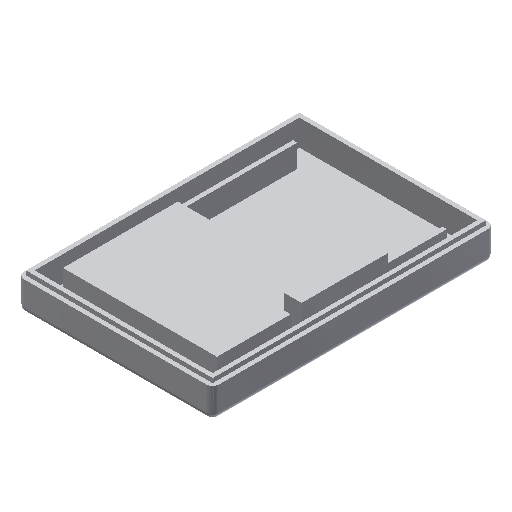
# Autodesk Inventor part: superior
Saved by Autodesk Inventor 2025.2 (Build 292293000, 293)
## iProperties
Created: 2025-10-19
Part Number: superior
Material: ABS Plastic
Document SubType Name: Sheet Metal
Designer: Ricardo
Density: 1.06 g/cm^3
Sheet Metal Rule: Default_mm
Appearance: Smooth - White
Mass: 10.1379 g
Surface Area: 106.906 cm^2
Volume: 9.56404 cm^3
Author: Ricardo
Autodesk Inventor part; units mm, degrees
ref_plane "YZ Plane" through (0, 0, 0) normal (1, 0, 0) x (0, 1, 0)
ref_plane "XZ Plane" through (0, 0, 0) normal (0, 1, 0) x (-1, 0, 0)
ref_plane "XY Plane" through (0, 0, 0) normal (0, 0, 1) x (1, 0, 0)
sketch "Sketch1" plane through (0, 0, 0) normal (0, 1, 0) x (-1, 0, 0)
  line L0 (0, 0) -> (45, 0)
  line L1 (45, 0) -> (45, -65)
  line L2 (45, -65) -> (0, -65)
  line L3 (0, -65) -> (0, 0)
  dimension "d0" = 45
  dimension "d1" = 65
  constraints: 8 end point, 2 parallel, 1 horizontal, 1 perpendicular
  measures "d0" distance of L1.end L2.end
  measures "d1" distance of L0.end L1.end
extrude "Extrusion1" add sketch "Sketch1" along normal blind 2
sketch "Sketch2" plane through (0, 2, 0) normal (0, 1, 0) x (1, 0, 0)
  line L0 (0, 65) -> (0, 0) projected
  line L1 (0, 0) -> (-45, 0) projected
  line L2 (-45, 0) -> (-45, 65) projected
  line L3 (-45, 65) -> (0, 65) projected
  line L4 (-45, 0) -> (0, 0) projected
  line L5 (-45, 65) -> (-45, 0) projected
  line L6 (0, 65) -> (-45, 65) projected
  line L7 (0, 0) -> (0, 65) projected
  line L8 (-2, 2) -> (-43, 2)
  line L9 (-43, 2) -> (-43, 63)
  line L10 (-43, 63) -> (-2, 63)
  line L11 (-2, 63) -> (-2, 2)
  dimension "d4" = 2
  dimension "d5" = 2
  dimension "d6" = 2
  dimension "d7" = 2
  constraints: 8 end point, 2 parallel, 1 horizontal, 1 perpendicular
  measures "d4" distance between parallel lines of L2 L9
  measures "d5" distance between parallel lines of L0 L11
  measures "d6" distance between parallel lines of L3 L10
  measures "d7" distance between parallel lines of L1 L8
extrude "Extrusion2" add sketch "Sketch2" along normal blind 2
sketch "Sketch3" plane through (0, 2, 0) normal (0, 1, 0) x (1, 0, 0)
  line L0 (-5.5, 6.5) -> (-39, 6.5)
  line L1 (-39, 6.5) -> (-39, 57.5)
  line L2 (-39, 57.5) -> (-5.5, 57.5)
  line L3 (-5.5, 57.5) -> (-5.5, 6.5)
  line L4 (0, 0) -> (0, 65) construction
  line L5 (0, 32.5) -> (-39, 32.5) construction
  line L6 (-45, 0) -> (0, 0) construction
  line L7 (-22.5, 0) -> (-22.5, 65) construction
  line L8 (0, 65) -> (-45, 65) construction
  line L9 (-4.5, 58.5) -> (-40, 58.5)
  line L10 (-40, 58.5) -> (-40, 5.5)
  line L11 (-40, 5.5) -> (-4.5, 5.5)
  line L12 (-4.5, 5.5) -> (-4.5, 58.5)
  line L13 (-2, 2) -> (-2, 63) projected
  line L14 (-2, 63) -> (-43, 63) projected
  line L15 (-43, 63) -> (-43, 2) projected
  line L16 (-43, 2) -> (-2, 2) projected
  line L17 (0, 65) -> (0, 0) projected
  line L18 (0, 0) -> (-45, 0) projected
  line L19 (-45, 0) -> (-45, 65) projected
  line L20 (-45, 65) -> (0, 65) projected
  dimension "d10" = 33.5
  dimension "d11" = 51
  dimension "d12" = 26
  dimension "d13" = 17
  dimension "d14" = 1
  dimension "d15" = 1
  dimension "d16" = 1
  dimension "d17" = 1
  dimension "d25" = 51
  constraints: 20 end point, 4 parallel, 3 midpoint, 3 perpendicular, 2 horizontal, 1 point on line
  measures "d10" distance of L1.end L2.end
  measures "d11" distance of L2.end L0.start
  measures "d12" distance between parallel lines of L0 L5
  measures "d13" distance between parallel lines of L7 L3
  measures "d14" distance between parallel lines of L3 L12
  measures "d15" distance between parallel lines of L11 L0
  measures "d16" distance between parallel lines of L1 L10
  measures "d17" distance between parallel lines of L2 L9
  measures "d25" distance of L0.end L1.end
extrude "Extrusion3" add sketch "Sketch3" along normal blind 5.25 contours L12 L11 L10 L9
sketch "Sketch4" plane through (-4.5, 2, -58.5) normal (0, 0, -1) x (-1, 0, 0)
  line L0 (35.5, 0) -> (0, 0) projected
  line L1 (35.5, 0) -> (35.5, 5.25) projected
  line L2 (0, 5.25) -> (35.5, 5.25) projected
  line L3 (0, 0) -> (0, 5.25) projected
  line L4 (1, 5.25) -> (34.5, 5.25)
  line L5 (34.5, 5.25) -> (34.5, 0)
  line L6 (34.5, 0) -> (1, 0)
  line L7 (1, 0) -> (1, 5.25)
  point P0 (-4.5, -2)
  point P1 (1, 0)
  point P2 (34.5, 0)
  dimension "d20" = 1
  dimension "d21" = 1
  dimension "d22" = 0
  constraints: 8 end point, 2 parallel, 1 horizontal, 1 perpendicular, 1 point on line
  measures "d20" distance between parallel lines of L3 L7
  measures "d21" distance between parallel lines of L1 L5
  measures "d22" distance between parallel lines of L0 L6
extrude "Extrusion4" cut sketch "Sketch4" against normal blind 2 contours L0 L7 L2 L5
sketch "Sketch5" plane through (0, 7.25, 0) normal (0, 1, 0) x (1, 0, 0)
  line L0 (-39, 58.5) -> (-39, 6.5) projected
  line L1 (-39, 6.5) -> (-5.5, 6.5) projected
  line L2 (-5.5, 6.5) -> (-5.5, 58.5) projected
  line L3 (-5.5, 58.5) -> (-4.5, 58.5) projected
  line L4 (-4.5, 58.5) -> (-4.5, 5.5) projected
  line L5 (-4.5, 5.5) -> (-40, 5.5) projected
  line L6 (-40, 5.5) -> (-40, 58.5) projected
  line L7 (-40, 58.5) -> (-39, 58.5) projected
  line L8 (-40, 5.5) -> (-4.5, 5.5)
  line L9 (-4.5, 5.5) -> (-4.5, 32)
  line L10 (-4.5, 32) -> (-40, 32)
  line L11 (-40, 32.75) -> (-40, 5.5)
  line L12 (-4.5, 32) -> (-40, 32)
  line L13 (-40, 32) -> (-40, 5.5)
  line L14 (-40, 5.5) -> (-4.5, 5.5)
  line L15 (-4.5, 5.5) -> (-4.5, 32)
  line L16 (-40, 58.5) -> (-40, 5.5) projected
  line L17 (-40, 5.5) -> (-4.5, 5.5) projected
  line L18 (-4.5, 5.5) -> (-4.5, 58.5) projected
  line L19 (-4.5, 32) -> (-40, 32)
  line L20 (-40, 32) -> (-40, 5.5)
  line L21 (-40, 5.5) -> (-4.5, 5.5)
  line L22 (-4.5, 5.5) -> (-4.5, 32.75)
  point P0 (0, 0)
  point P1 (-5.5, 32)
  point P2 (-39, 32)
  constraints: 24 end point, 5 parallel, 3 perpendicular, 2 horizontal, 1 midpoint
extrude "Extrusion6" add sketch "Sketch5" along normal blind 1 contours L10 L2 L1 L0 | L0 L1 L2 L10 L4 L5 L6
fillet "Fillet1" radius 1.5 1 edges at (-22.5, 0, 0)
fillet "Fillet2" radius 1.5 1 edges at (-22.5, 0, -65)
sketch "Sketch13" plane through (0, 8.25, 0) normal (0, 1, 0) x (1, 0, 0)
  line L0 (0, 0) -> (0, 65) projected
  line L1 (-4.5, 5.5) -> (-4.5, 32) projected
  line L2 (-4.5, 32) -> (-4.5, 58.5) projected
  line L3 (-5.5, 6.5) -> (-5.5, 58.5) projected
  line L4 (-40, 32) -> (-40, 5.5) construction
  line L5 (-40, 5.5) -> (-4.5, 5.5) construction
  line L6 (-4.5, 5.5) -> (-4.5, 32) construction
  line L7 (-4.5, 32) -> (-40, 32) construction
  line L8 (-2, 63) -> (-2, 2) projected
  line L9 (-40, 5.5) -> (-4.5, 5.5) projected
  line L10 (-4.5, 32) -> (-40, 32) projected
  line L11 (-2, 42.5) -> (-6, 42.5)
  line L12 (-6, 42.5) -> (-6, 22.5)
  line L13 (-6, 22.5) -> (-2, 22.5)
  line L14 (-2, 22.5) -> (-2, 42.5)
  line L15 (-2, 2) -> (-43, 2) projected
  point P0 (-5.75, 59.75)
  point P1 (-4.5, 22.5)
  point P2 (-2, 22.5)
  point P3 (-4.5, 42.5)
  dimension "d58" = 4
  dimension "d59" = 20
  dimension "d60" = 20.5
  constraints: 8 end point, 2 parallel, 1 horizontal, 1 perpendicular, 1 point on line, 1 other
  measures "d58" distance of L13.end L12.end
  measures "d59" distance of L11.end L12.end
  measures "d60" distance between parallel lines of L15 L13
extrude "Extrusion12" add sketch "Sketch13" along normal mid plane 7
sketch "Sketch15" plane through (-2, 11.75, -42.5) normal (0, 0, -1) x (-1, 0, 0)
  line L0 (4, -3.5) -> (38, -3.5) projected
  line L1 (4, -4.5) -> (37, -4.5) projected
  line L2 (3.5, -7) -> (3.5, -4.5) projected
  line L3 (37, -9.75) -> (3.5, -9.75) projected
  line L4 (3.5, -4.5) -> (4, -4.5)
  line L5 (4, -4.5) -> (4, -13.75)
  line L6 (4, -13.75) -> (3.5, -13.75)
  line L7 (3.5, -13.75) -> (3.5, -4.5)
  point P0 (-2, -11.75)
  point P1 (3.5, -13.75)
  point P2 (4, -9.75)
  constraints: 8 end point, 2 parallel, 1 horizontal, 1 perpendicular, 1 other
extrude "Extrusion14" cut sketch "Sketch15" against normal up to surface (36 mm away) contours L2 L4 L5 L3 L7
sketch "Sketch16" plane through (0, 4, 0) normal (0, 1, 0) x (1, 0, 0)
  line L0 (-2, 22.5) -> (-2, 42.5) projected
  line L1 (-2, 22.5) -> (-2, 2) projected
  line L2 (-2, 2) -> (-43, 2) projected
  line L3 (-45, 0) -> (0, 0) projected
  line L4 (0, 0) -> (0, 65) projected
  line L5 (-2, 63) -> (-2, 42.5) projected
  line L6 (-43, 63) -> (-2, 63) projected
  line L7 (0, 65) -> (-45, 65) projected
  line L8 (-45, 65) -> (-45, 0) projected
  line L9 (-43, 2) -> (-43, 63) projected
  line L10 (0, 65) -> (-45, 65)
  line L11 (-45, 65) -> (-45, 0)
  line L12 (-45, 0) -> (0, 0)
  line L13 (0, 0) -> (0, 65)
  line L14 (-43, 2) -> (-2, 2)
  line L15 (-2, 2) -> (-2, 63)
  line L16 (-2, 63) -> (-43, 63)
  line L17 (-43, 63) -> (-43, 2)
  constraints: 16 end point, 4 parallel, 2 horizontal, 2 perpendicular
extrude "Extrusion15" add sketch "Sketch16" along normal blind 4
sketch "Sketch17" plane through (0, 8, 0) normal (0, 1, 0) x (1, 0, 0)
  line L0 (0, 0) -> (0, 65) projected
  line L1 (0, 65) -> (-45, 65) projected
  line L2 (-45, 0) -> (0, 0) projected
  line L3 (-45, 65) -> (-45, 0) projected
  line L4 (-1, 64) -> (-44, 64)
  line L5 (-44, 64) -> (-44, 1)
  line L6 (-44, 1) -> (-1, 1)
  line L7 (-1, 1) -> (-1, 64)
  dimension "d71" = 1
  dimension "d72" = 1
  dimension "d73" = 1
  dimension "d74" = 1
  constraints: 8 end point, 2 parallel, 1 horizontal, 1 perpendicular
  measures "d71" distance between parallel lines of L2 L6
  measures "d72" distance between parallel lines of L0 L7
  measures "d73" distance between parallel lines of L1 L4
  measures "d74" distance between parallel lines of L5 L3
extrude "Extrusion16" cut sketch "Sketch17" against normal blind 1
fillet "Fillet3" radius 1.5 5 edges at (0, 0.4393, -0.4393) (0, 0, -32.5) (0, 0.4393, -64.5607) (0, 4.25, -65) (0, 4.25, 0)
fillet "Fillet4" radius 1.5 5 edges at (-45, 0.4393, -0.4393) (-45, 4.25, 0) (-45, 0.4393, -64.5607) (-45, 4.25, -65) (-45, 0, -32.5)
equation "\"BendRadius\" = Thickness"
equation "\"BendReliefWidth\" = Thickness"
equation "\"BendReliefDepth\" = 0.5 * Thickness"
equation "\"CornerReliefSize\" = 4 * Thickness"
equation "\"MinimumRemnant\" = 2 * Thickness"
equation "\"TransitionRadius\" = BendRadius"
equation "\"JacobiRadiusSize\" = BendRadius"
equation "\"GapSize\" = Thickness"
equation "\"Thickness\" = 0.5"
body "Solid1"
